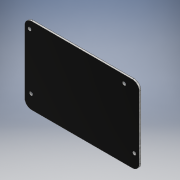
# Autodesk Inventor part: Teensy And Breakout
Saved by Autodesk Inventor 2018 (Build 220112000, 112)
## iProperties
Created: 2018-09-04
Part Number: Teensy And Breakout
Material: Generic
Document SubType Name: Modeling
Designer: matth
Density: 1 g/cm^3
Appearance: Default
Author: matth
Autodesk Inventor part; units mm, degrees
ref_plane "YZ Plane" through (0, 0, 0) normal (1, 0, 0) x (0, 1, 0)
ref_plane "XZ Plane" through (0, 0, 0) normal (0, 1, 0) x (-1, 0, 0)
ref_plane "XY Plane" through (0, 0, 0) normal (0, 0, 1) x (1, 0, 0)
sketch "Sketch1" plane through (0, 0, 0) normal (0, 1, 0) x (-1, 0, 0)
  line L0 (0, 0) -> (-4.3, 0)
  line L1 (-4.3, 0) -> (-4.3, -12)
  line L2 (-4.3, -12) -> (95.7, -12)
  line L3 (95.7, -12) -> (95.7, 55)
  line L4 (95.7, 55) -> (-4.3, 55)
  line L5 (-4.3, 55) -> (-4.3, 0)
  circle A0 centre (0, 0) radius 1.5
  line L6 (0, 0) -> (90.17, 0)
  circle A1 centre (90.17, 0) radius 1.5
  line L7 (-4.3, 55) -> (-4.3, 48.26)
  line L8 (-4.3, 48.26) -> (8.89, 48.26)
  line L9 (8.89, 48.26) -> (91.44, 48.26)
  circle A2 centre (8.89, 48.26) radius 1.5
  circle A3 centre (91.44, 48.26) radius 1.5
  dimension "d0" = 4.3
  dimension "d1" = 12
  dimension "d2" = 100
  dimension "d3" = 67
  dimension "d4" = 3
  dimension "d5" = 90.17
  dimension "d6" = 3
  dimension "d7" = 6.74
  dimension "d8" = 13.19
  dimension "d9" = 82.55
  dimension "d10" = 3
  dimension "d11" = 3
  constraints: 20 end point, 4 centre point, 4 coincident, 4 horizontal, 4 perpendicular, 1 point on line, 1 vertical
  measures "d0" distance of L0.start L0.end
  measures "d1" distance of L0.end L1.end
  measures "d2" distance of L1.end L2.end
  measures "d3" distance of L2.end L3.end
  measures "d4" diameter of A0
  measures "d5" distance of L6.start L6.end
  measures "d6" diameter of A1
  measures "d7" distance of L4.end L7.end
  measures "d8" distance of L7.end L8.end
  measures "d9" distance of L8.end L9.end
  measures "d10" diameter of A2
  measures "d11" diameter of A3
extrude "Extrusion1" add sketch "Sketch1" along normal blind 1.5
fillet "Fillet1" radius 6 4 edges at (-95.7, 0.75, 55) (-95.7, 0.75, -12) (4.3, 0.75, -12) (4.3, 0.75, 55)
sketch "Sketch3" plane through (0, 1.5, 0) normal (0, 1, 0) x (1, 0, 0)
  line L0 (-80.2385, -43.3473) -> (-35.2385, -43.3473)
  line L1 (-35.2385, -43.3473) -> (-35.2385, -23.3473)
  line L2 (-35.2385, -23.3473) -> (-80.2385, -23.3473)
  line L3 (-80.2385, -23.3473) -> (-80.2385, -43.3473)
  line L4 (-35.2385, -43.3473) -> (-80.2385, -43.3473)
  line L5 (-80.2385, -43.3473) -> (-80.2385, -39.3473)
  line L6 (-80.2385, -39.3473) -> (-35.2385, -39.3473)
  line L7 (-35.2385, -39.3473) -> (-35.2385, -43.3473)
  line L8 (-35.2385, -23.3473) -> (-80.2385, -23.3473)
  line L9 (-80.2385, -23.3473) -> (-80.2385, -27.3473)
  line L10 (-80.2385, -27.3473) -> (-35.2385, -27.3473)
  line L11 (-35.2385, -27.3473) -> (-35.2385, -23.3473)
  point P0 (0, 0)
  dimension "d15" = 45
  dimension "d16" = 20
  dimension "d17" = 4
  dimension "d18" = 4
  constraints: 24 end point, 6 parallel, 3 horizontal, 3 perpendicular, 2 point on line
  measures "d15" distance of L2.end L1.end
  measures "d16" distance of L1.end L0.end
  measures "d17" distance of L4.end L5.end
  measures "d18" distance of L9.end L8.end
extrude "Extrusion2" add sketch "Sketch3" along normal blind 8 contours L3 L6 L1 L0 | L3 L2 L1 L10
sketch "Sketch4" plane through (0, 9.5, 0) normal (0, 1, 0) x (1, 0, 0)
  line L0 (-80.2385, -39.3473) -> (-80.2385, -43.3473) projected
  line L1 (-80.2385, -43.3473) -> (-81.2385, -43.3473)
  line L2 (-81.2385, -43.3473) -> (-81.2385, -44.3473)
  line L3 (-81.2385, -44.3473) -> (-34.2385, -44.3473)
  line L4 (-34.2385, -44.3473) -> (-34.2385, -22.3473)
  line L5 (-34.2385, -22.3473) -> (-81.2385, -22.3473)
  line L6 (-81.2385, -22.3473) -> (-81.2385, -44.3473)
  point P0 (0, 0)
  dimension "d21" = 1
  dimension "d22" = 1
  dimension "d23" = 47
  dimension "d24" = 22
  constraints: 12 end point, 2 horizontal, 2 parallel, 2 perpendicular
  measures "d21" distance of L0.end L1.end
  measures "d22" distance of L1.end L2.end
  measures "d23" distance of L5.end L4.end
  measures "d24" distance of L4.end L3.end
extrude "Extrusion3" add sketch "Sketch4" along normal blind 1.5
sketch "Sketch5" plane through (0, 11, 0) normal (0, 1, 0) x (1, 0, 0)
  line L0 (-81.2385, -22.3473) -> (-81.2385, -44.3473) projected
  line L1 (-81.2385, -33.3473) -> (-76.2385, -33.3473)
  line L2 (-76.2385, -33.3473) -> (-76.2385, -31.3473)
  line L3 (-76.2385, -31.3473) -> (-81.2385, -31.3473)
  line L4 (-81.2385, -31.3473) -> (-81.2385, -33.3473)
  line L5 (-81.2385, -33.3473) -> (-76.2385, -33.3473)
  line L6 (-76.2385, -33.3473) -> (-76.2385, -35.3473)
  line L7 (-76.2385, -35.3473) -> (-81.2385, -35.3473)
  line L8 (-81.2385, -35.3473) -> (-81.2385, -33.3473)
  line L9 (-34.2385, -44.3473) -> (-34.2385, -22.3473) projected
  line L10 (-34.2385, -33.3473) -> (-36.2385, -33.3473)
  line L11 (-36.2385, -33.3473) -> (-36.2385, -29.3473)
  line L12 (-36.2385, -29.3473) -> (-34.2385, -29.3473)
  line L13 (-34.2385, -29.3473) -> (-34.2385, -33.3473)
  line L14 (-36.2385, -29.3473) -> (-44.2385, -29.3473)
  line L15 (-44.2385, -29.3473) -> (-44.2385, -37.3473)
  line L16 (-44.2385, -37.3473) -> (-36.2385, -37.3473)
  line L17 (-36.2385, -37.3473) -> (-36.2385, -29.3473)
  point P0 (0, 0)
  dimension "d27" = 5
  dimension "d28" = 2
  dimension "d29" = 2
  dimension "d30" = 2
  dimension "d31" = 4
  dimension "d32" = 8
  dimension "d33" = 8
  constraints: 32 end point, 8 parallel, 4 horizontal, 4 perpendicular, 2 midpoint
  measures "d27" distance of L3.end L2.end
  measures "d28" distance of L2.end L1.end
  measures "d29" distance of L5.end L6.end
  measures "d30" distance of L11.end L12.end
  measures "d31" distance of L10.end L11.end
  measures "d32" distance of L16.end L15.end
  measures "d33" distance of L15.end L14.end
extrude "Extrusion4" add sketch "Sketch5" along normal blind 3 contours L3 L2 L1 L0 | L1 L6 L7 L0 | L17 L16 L15 L14 L11
sketch "Sketch6" plane through (-81.2385, 9.5, 22.3473) normal (-1, 0, 0) x (0, 0, 1)
  line L0 (13, 1.5) -> (13, 4.5) projected
  line L1 (9, 1.5) -> (9, 4.5) projected
  line L2 (13, 4.5) -> (9, 4.5)
  line L3 (9, 4.5) -> (9, 1.5)
  line L4 (9, 1.5) -> (13, 1.5)
  line L5 (13, 1.5) -> (13, 4.5)
  point P0 (-22.3473, -9.5)
  constraints: 8 end point, 2 parallel, 1 horizontal, 1 perpendicular
extrude "Extrusion5" cut sketch "Sketch6" against normal blind 0.01
body "Solid1"
